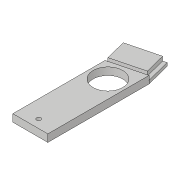
# Autodesk Inventor part: Lidar Sensor Case Piece 2
Saved by Autodesk Inventor 2018.3 (Build 223284000, 284)
## iProperties
Created: 2019-02-26
Part Number: Lidar Sensor Case Piece 2
Material: Generic
Document SubType Name: Modeling
Designer: aye06091
Mass: 11.1601 g
Surface Area: 60.4599 cm^2
Volume: 11.1601 cm^3
Density: 1 g/cm^3
Appearance: Default
Author: aye06091
Autodesk Inventor part; units mm, degrees
ref_plane "YZ Plane" through (0, 0, 0) normal (1, 0, 0) x (0, 1, 0)
ref_plane "XZ Plane" through (0, 0, 0) normal (0, 1, 0) x (-1, 0, 0)
ref_plane "XY Plane" through (0, 0, 0) normal (0, 0, 1) x (1, 0, 0)
sketch "Sketch1" plane through (0, 0, 0) normal (0, 1, 0) x (-1, 0, 0)
  line L0 (18.6455, 5.0782) -> (18.6456, 5.0782)
  line L1 (-34.5212, -26.5719) -> (-29.8086, -45.0298)
  line L2 (-29.8086, -45.0298) -> (-3.3186, -38.2664)
  circle A0 centre (-21.2762, -8.696) radius 11.176
  line L3 (-8.0312, 50.0415) -> (-8.0312, -19.8085)
  line L4 (-8.0312, -19.8085) -> (-3.3186, -38.2664)
  line L5 (-3.3186, -38.2664) -> (-29.8086, -45.0298)
  line L6 (-29.8086, -45.0298) -> (-34.5212, -26.5719)
  line L7 (-34.5212, -26.5719) -> (-34.5212, 50.0415)
  line L8 (-8.0312, 50.0415) -> (-34.5212, 50.0415)
  point P0 (0, 0)
  dimension "d4" = 22.352
  dimension "d24" = 19.05
  dimension "d25" = 69.85
  dimension "d26" = 19.05
  dimension "d28" = 26.49
  dimension "d29" = 13.245
  dimension "d35" = 58.7375
  dimension "d36" = 75.677
  constraints: 18 end point, 4 perpendicular, 1 centre point, 1 parallel, 1 vertical
  measures "d4" diameter of A0
  measures "d24" distance of L3.end L2.end
  measures "d25" distance of L3.start L3.end
  measures "d26" distance of L1.start L1.end
  measures "d28" distance of L3.start L7.end
  measures "d29" distance from line of L7 A0.centre
  measures "d35" distance from line of L8 A0.centre
  measures "d36" angle of L7 L2
extrude "Extrusion1" add sketch "Sketch1" along normal blind 5.6134
sketch "Sketch2" plane through (0, 5.6134, 0) normal (0, 1, 0) x (1, 0, 0)
  line L0 (34.5212, 26.5719) -> (29.8086, 45.0298) projected
  line L1 (8.0312, 19.8085) -> (34.5212, 26.5719)
  line L2 (34.5212, 26.5719) -> (33.7735, 29.5006)
  line L3 (33.7735, 29.5006) -> (7.2835, 22.7372)
  line L4 (7.2835, 22.7372) -> (8.0312, 19.8085)
  point P0 (0, 0)
  point P1 (0, 0)
  dimension "d37" = 3.0226
  constraints: 8 end point, 2 parallel, 1 perpendicular
  measures "d37" distance of L2.end L0.start
extrude "Extrusion2" cut sketch "Sketch2" against normal blind 3.175
sketch "Sketch3" plane through (0, 5.6134, 0) normal (0, 1, 0) x (1, 0, 0)
  line L0 (33.7735, 29.5006) -> (29.8086, 45.0298) projected
  line L1 (29.8086, 45.0298) -> (3.3186, 38.2664) projected
  line L2 (29.8086, 45.0298) -> (34.5212, 26.5719) projected
  line L3 (29.8086, 45.0298) -> (34.5212, 26.5719)
  line L4 (34.5212, 26.5719) -> (31.8018, 25.8776)
  line L5 (31.8018, 25.8776) -> (27.0891, 44.3355)
  line L6 (27.0891, 44.3355) -> (29.8086, 45.0298)
  point P0 (0, 0)
  point P1 (27.0891, 44.3355)
  dimension "d38" = 2.8067
  constraints: 8 end point, 3 equal length, 1 perpendicular, 1 point on line
  measures "d38" distance between parallel lines of L0 L5
extrude "Extrusion3" cut sketch "Sketch3" against normal blind 3.175
sketch "Sketch4" plane through (0, 5.6134, 0) normal (0, 1, 0) x (1, 0, 0)
  line L0 (8.0312, -50.0415) -> (34.5212, -50.0415) projected
  line L1 (34.5212, -50.0415) -> (34.5212, 26.5719) projected
  circle A0 centre (21.2762, -43.6915) radius 1.6002
  point P0 (0, 0)
  dimension "d30" = 3.2004
  dimension "d31" = 13.245
  dimension "d32" = 6.35
  constraints: 1 centre point
  measures "d30" diameter of A0
  measures "d31" distance from line of L1 A0.centre
  measures "d32" distance from line of L0 A0.centre
extrude "Extrusion4" cut sketch "Sketch4" against normal blind 25.4
body "Solid1"
